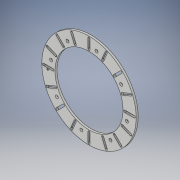
# Autodesk Inventor part: anillo bajo
Saved by Autodesk Inventor 2019 (Build 230136000, 136)
## iProperties
Created: 2020-02-07
Part Number: anillo bajo
Material: Generic
Document SubType Name: Modeling
Designer: Hugo Albarracin
Density: 1 g/cm^3
Appearance: Default
Author: Hugo Albarracin
Autodesk Inventor part; units mm, degrees
sketch "Sketch1" plane through (0, 0, 0) normal (0, 0, 1) x (1, 0, 0)
  circle A0 centre (0, 0) radius 120
  circle A1 centre (0, 0) radius 88
  dimension "d0" = 240
  dimension "d90" = 32
  constraints: 2 centre point, 2 coincident
  measures "d0" diameter of A0
  measures "d90" radial gap between concentric circles of A0 A1
extrude "Extrusion1" add sketch "Sketch1" along normal blind 5.2
sketch "Sketch2" plane through (0, 0, 5.2) normal (0, 0, 1) x (1, 0, 0)
  circle A0 centre (0, 0) radius 120 construction
  line L0 (-125, 0) -> (-88.9843, 0) construction
  line L1 (-88.0046, 2.1786) -> (-87.973, 2.1786)
  circle A1 centre (-120, 0) radius 2.75 construction
  circle A2 centre (-90, 0) radius 2.75 construction
  arc A3 (-117.25, 2.75) -> (-117.25, -2.75) centre (-117.25, 0) ccw
  arc A4 (-90, 0) -> (-90, 0) centre (-92.75, 0) ccw
  line L2 (-88.9843, 0) -> (0, 0) construction
  line L3 (-117.25, -2.75) -> (-117.25, 0) construction
  line L4 (-117.25, 2.75) -> (-117.25, 0) construction
  arc A5 (-92.75, -2.75) -> (-92.75, 2.75) centre (-92.75, 0) ccw
  line L5 (-117.25, -2.75) -> (-92.75, -2.75)
  line L6 (-117.25, 2.75) -> (-92.75, 2.75)
  line L7 (-92.75, 2.75) -> (-92.75, -2.75) construction
  dimension "d29" = 5.5
  dimension "d30" = 5.5
  dimension "d22" = 125
  dimension "d31" = 5.5
  dimension "d91" = 90
  constraints: 16 end point, 7 point on circle, 4 horizontal, 4 point on line, 3 centre point, 3 horizontal alignment, 3 vertical, 1 coincident, 1 collinear, 1 tangent, 5 other
  measures "d22" distance of point (0, 0) L0.start
  measures "d31" diameter of A3
  measures "d91" distance of point (0, 0) A4.start
extrude "Extrusion3" cut sketch "Sketch2" against normal through all
pattern_circular "Circular Pattern2" count 16 over 360 about axis through (0, 0, 0) along (0, 0, 1) of "Extrusion3"
ref_plane "Work Plane1" through (0, 0, 2.6) normal (0, 0, 1) x (1, 0, 0)
sketch "Sketch3" plane through (0, 0, 2.6) normal (0, 0, 1) x (1, 0, 0)
  circle A0 centre (0, 0) radius 122
  circle A1 centre (0, 0) radius 120
  arc A2 (-120, 0) -> (-110.8655, -45.922) centre (0, 0) ccw projected
  arc A3 (-120, 0) -> (-110.8655, -45.922) centre (0, 0) ccw projected
  arc A4 (-110.8655, -45.922) -> (-84.8528, -84.8528) centre (0, 0) ccw projected
  arc A5 (-110.8655, -45.922) -> (-84.8528, -84.8528) centre (0, 0) ccw projected
  arc A6 (84.8528, -84.8528) -> (110.8655, -45.922) centre (0, 0) ccw projected
  arc A7 (84.8528, -84.8528) -> (110.8655, -45.922) centre (0, 0) ccw projected
  arc A8 (-84.8528, -84.8528) -> (-45.922, -110.8655) centre (0, 0) ccw projected
  arc A9 (-84.8528, -84.8528) -> (-45.922, -110.8655) centre (0, 0) ccw projected
  arc A10 (-45.922, -110.8655) -> (0, -120) centre (0, 0) ccw projected
  arc A11 (-45.922, -110.8655) -> (0, -120) centre (0, 0) ccw projected
  arc A12 (0, -120) -> (45.922, -110.8655) centre (0, 0) ccw projected
  arc A13 (0, -120) -> (45.922, -110.8655) centre (0, 0) ccw projected
  arc A14 (45.922, -110.8655) -> (84.8528, -84.8528) centre (0, 0) ccw projected
  arc A15 (45.922, -110.8655) -> (84.8528, -84.8528) centre (0, 0) ccw projected
  arc A16 (120, 0) -> (110.8655, 45.922) centre (0, 0) ccw projected
  arc A17 (120, 0) -> (110.8655, 45.922) centre (0, 0) ccw projected
  arc A18 (110.8655, -45.922) -> (120, 0) centre (0, 0) ccw projected
  arc A19 (110.8655, -45.922) -> (120, 0) centre (0, 0) ccw projected
  arc A20 (-110.8655, 45.922) -> (-120, 0) centre (0, 0) ccw projected
  arc A21 (-110.8655, 45.922) -> (-120, 0) centre (0, 0) ccw projected
  arc A22 (110.8655, 45.922) -> (84.8528, 84.8528) centre (0, 0) ccw projected
  arc A23 (110.8655, 45.922) -> (84.8528, 84.8528) centre (0, 0) ccw projected
  arc A24 (84.8528, 84.8528) -> (45.922, 110.8655) centre (0, 0) ccw projected
  arc A25 (84.8528, 84.8528) -> (45.922, 110.8655) centre (0, 0) ccw projected
  arc A26 (45.922, 110.8655) -> (0, 120) centre (0, 0) ccw projected
  arc A27 (45.922, 110.8655) -> (0, 120) centre (0, 0) ccw projected
  arc A28 (0, 120) -> (-45.922, 110.8655) centre (0, 0) ccw projected
  arc A29 (0, 120) -> (-45.922, 110.8655) centre (0, 0) ccw projected
  arc A30 (-45.922, 110.8655) -> (-84.8528, 84.8528) centre (0, 0) ccw projected
  arc A31 (-45.922, 110.8655) -> (-84.8528, 84.8528) centre (0, 0) ccw projected
  arc A32 (-84.8528, 84.8528) -> (-110.8655, 45.922) centre (0, 0) ccw projected
  arc A33 (-84.8528, 84.8528) -> (-110.8655, 45.922) centre (0, 0) ccw projected
  dimension "d97" = 244
  dimension "d98" = 240
  constraints: 2 centre point
  measures "d97" diameter of A0
  measures "d98" diameter of A1
extrude "Extrusion5" add sketch "Sketch3" along normal mid plane 5.2
sketch "Sketch5" plane through (0, 0, 5.2) normal (0, 0, 1) x (1, 0, 0)
  line L0 (0, 0) -> (-89.8964, 0) construction
  line L1 (0, 0) -> (-98.0785, 19.509) construction
  circle A0 centre (-98.0785, 19.509) radius 2.5 construction
  circle A1 centre (0, 0) radius 88 construction
  circle A2 centre (0, 0) radius 100 construction
  dimension "d45" = 11.25
  dimension "d46" = 5
  dimension "d95" = 12
  constraints: 4 end point, 2 coincident, 1 centre point, 1 horizontal, 3 other
  measures "d45" angle of L1 L0
  measures "d46" diameter of A0
ref_plane "Work Plane2" through (0, 0, 5.2) normal (0.1950903, 0.9807853, 0) x (-0.9807853, 0.1950903, 0)
sketch "Sketch9" plane through (0, 0, 5.2) normal (0.1950903, 0.9807853, 0) x (-0.9807853, 0.1950903, 0)
  line L0 (102.5, 0) -> (97.5, 0) construction
  line L1 (100, 0) -> (100, -5.2)
  line L2 (102, -5.2) -> (102, -3.1)
  line L3 (100, 0) -> (104, 0)
  line L4 (104, 0) -> (102, -3.1)
  line L5 (-122, -5.2) -> (122, -5.2) construction
  line L6 (102, -5.2) -> (100, -5.2)
  point P0 (0, -5.2)
  dimension "d65" = 4
  dimension "d66" = 3.1
  dimension "d96" = 2
  constraints: 10 end point, 2 vertical, 1 collinear, 1 horizontal, 1 midpoint
  measures "d65" distance of L1.start L3.end
  measures "d66" distance from line of L3 L2.end
  measures "d96" distance between parallel lines of L1 L2
revolve "Revolution2" cut sketch "Sketch9" angle 360 about axis through (-98.0785, 19.509, 5.2) along (0, 0, -1)
pattern_circular "Circular Pattern4" count 8 over 360 about axis through (0, 0, 0) along (0, 0, 1) of "Revolution2"
sketch "Sketch10" plane through (0, 0, 5.2) normal (0, 0, 1) x (1, 0, 0)
  line L0 (0, 0) -> (-140, 0) construction
  line L1 (0, 0) -> (-21.2891, 85.386)
  circle A0 centre (0, 0) radius 140
  arc A1 (122, 0) -> (122, 0) centre (0, 0) ccw projected
  circle A2 centre (0, 0) radius 88 projected
  line L2 (-29.5145, 118.3761) -> (-33.8691, 135.8414)
  arc A3 (-26.6114, 106.7325) -> (-24.676, 98.9702) centre (-25.6437, 102.8513) ccw construction
  line L3 (-21.7599, 107.9421) -> (-19.8246, 100.1798)
  line L4 (-26.6114, 106.7325) -> (-21.7599, 107.9421)
  line L5 (-24.676, 98.9702) -> (-19.8246, 100.1798)
  line L6 (-21.2891, 85.386) -> (-24.676, 98.9702)
  line L7 (-26.6114, 106.7325) -> (-29.5145, 118.3761)
  line L8 (121.3317, -12.7525) -> (139.2331, -14.634)
  arc A4 (109.3974, -11.4981) -> (101.4412, -10.6619) centre (105.4193, -11.08) ccw construction
  line L9 (108.8748, -16.4707) -> (100.9186, -15.6345)
  line L10 (109.3974, -11.4981) -> (108.8748, -16.4707)
  line L11 (101.4412, -10.6619) -> (100.9186, -15.6345)
  line L12 (89.507, -9.4076) -> (101.4412, -10.6619)
  line L13 (109.3974, -11.4981) -> (121.3317, -12.7525)
  line L14 (0, 0) -> (89.507, -9.4076)
  line L15 (-56.6542, -94.2884) -> (-62.8346, -104.5744)
  line L16 (-56.6542, -94.2884) -> (-60.94, -91.7132)
  arc A5 (-56.6542, -94.2884) -> (-52.5339, -87.4311) centre (-54.594, -90.8597) ccw construction
  line L17 (-60.94, -91.7132) -> (-56.8197, -84.8559)
  line L18 (-52.5339, -87.4311) -> (-56.8197, -84.8559)
  line L19 (-46.3534, -77.1451) -> (-52.5339, -87.4311)
  line L20 (-62.8346, -104.5744) -> (-72.1053, -120.0034)
  line L21 (0, 0) -> (-46.3534, -77.1451)
  dimension "d74" = 140
  dimension "d75" = 140
  dimension "d76" = 76
  dimension "d83" = 8
  dimension "d86" = 8
  dimension "d88" = 110
  dimension "d89" = 8
  constraints: 44 end point, 7 point on circle, 6 tangent, 3 centre point, 3 perpendicular, 2 coincident, 1 horizontal, 5 other
  measures "d74" distance of L0.start L0.end
  measures "d75" distance of L0.start L2.end
  measures "d76" angle of L1 L0
  measures "d83" diameter of A3
  measures "d86" diameter of A4
  measures "d88" angle of L1 L14
  measures "d89" diameter of A5
sketch "Sketch13" plane through (0, 0, 5.2) normal (0, 0, 1) x (1, 0, 0)
  circle A0 centre (-106.8707, -6.0513) radius 2.1161
  point P0 (0, 0)
  constraints: 1 centre point
extrude "Extrusion8" cut sketch "Sketch13" against normal blind 1
ref_plane "Work Plane4" through (-117.25, 0, 5.2) normal (0, -1, 0) x (1, 0, 0)
equation "\"d0\" = diametro_max"
equation "\"d30\" = d29"
equation "\"d31\" = d29"
equation "\"d36\" = d3"
equation "\"angulo_alabe\" = 130deg"
equation "\"diametro_max\" = 240"
equation "\"d24\" = 0.5 * d25"
equation "\"diametro_tubo\" = 232"
equation "\"d32\" = d29"
equation "\"desfase_pin_superior\" = 12"
equation "\"desfase_b_pin_inferior\" = 8"
equation "\"desfase_b_pin_superior\" = 0"
equation "\"desfase_a_pin_superior\" = 12"
equation "\"diametro_max_soporte\" = 248"
equation "\"d3\" = 5.2"
equation "\"d25\" = 5.1"
body "Solid1"
